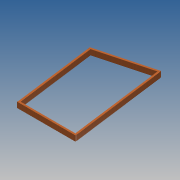
# Autodesk Inventor part: H7jp.E_UfaA-panelEframe
Saved by Autodesk Inventor 2014 SP1 (Build 180222100, 222)
## iProperties
Company: HERA
Created: 2015-04-29
Part Number: H7jp.E_UfaA-panelEframe
Material: Wood (Cherry)
Document SubType Name: Modeling
Designer: Dave
Mass: 16881.5 g
Surface Area: 18802.7 cm^2
Volume: 26796 cm^3
Density: 0.63 g/cm^3
Appearance: Cherry - Natural Low Gloss
Title: HERA Panel E frame
Author: Dave
Revision Number: A
Autodesk Inventor part; units mm, degrees
ref_plane "YZ Plane" through (0, 0, 0) normal (1, 0, 0) x (0, 1, 0)
ref_plane "XZ Plane" through (0, 0, 0) normal (0, 1, 0) x (-1, 0, 0)
ref_plane "XY Plane" through (0, 0, 0) normal (0, 0, 1) x (1, 0, 0)
sketch "Sketch1" plane through (0, 0, 0) normal (0, 1, 0) x (-1, 0, 0)
  line L0 (-1224.9972, -38) -> (-960.8978, -2044.0342)
  line L1 (-951.0627, -2080.7394) -> (232.1938, -1763.6868)
  line L2 (-955.895, -2082.0342) -> (274.105, -2082.0342) construction
  line L3 (227.191, -1725.6868) -> (5.0028, -38)
  line L4 (190.1691, -1735.6068) -> (-33.3251, -38)
  line L5 (-33.3251, -38) -> (-1186.6693, -38)
  line L6 (-1186.6693, -38) -> (-923.8759, -2034.1142)
  line L7 (-960.8978, -2044.0342) -> (-951.0627, -2080.7394)
  line L8 (-923.8759, -2034.1142) -> (190.1691, -1735.6068)
  line L9 (-1224.9972, -38) -> (-1224.9972, 0)
  line L10 (5.0028, -38) -> (5.0028, 0)
  line L11 (-1230, 0) -> (-1224.9972, 0) construction
  line L12 (5.0028, 0) -> (870, 0) construction
  line L13 (5.0028, 0) -> (-1224.9972, 0)
  line L14 (232.1938, -1763.6868) -> (237.0261, -1762.392)
  line L15 (227.191, -1725.6868) -> (237.0261, -1762.392)
  dimension "d1" = 2100
  dimension "d9" = 1230
  dimension "d10" = 15
  dimension "d12" = 38
  constraints: 32 end point, 4 perpendicular, 3 horizontal, 1 collinear, 1 parallel
  measures "d1" distance of L11.start L2.start
  measures "d9" distance of L2.start L1.end
  measures "d10" angle of L2 L1
  measures "d12" distance between parallel lines of L6 L0
extrude "Extrusion1" add sketch "Sketch1" along normal blind 114
sketch "Sketch2" plane through (0, 114, 0) normal (0, 1, 0) x (1, 0, 0)
  line L0 (33.3251, 38) -> (-190.1691, 1735.6068) projected
  line L1 (-227.191, 1725.6868) -> (-5.0028, 38) projected
  line L2 (1224.9972, 0) -> (1224.9972, 38) projected
  line L3 (960.8978, 2044.0342) -> (951.0627, 2080.7394) projected
  line L4 (-190.1691, 1735.6068) -> (-227.191, 1725.6868)
  line L5 (33.3251, 38) -> (-5.0028, 38)
  point P0 (0, 0)
  constraints: 4 end point, 2 perpendicular
extrude "Extrusion2" cut sketch "Sketch2" against normal blind 1
sketch "Sketch3" plane through (0, 114, 0) normal (0, 1, 0) x (1, 0, 0)
  line L0 (1224.9972, 0) -> (1224.9972, 38) projected
  line L1 (1224.9972, 38) -> (960.8978, 2044.0342) projected
  line L2 (960.8978, 2044.0342) -> (951.0627, 2080.7394) projected
  line L3 (951.0627, 2080.7394) -> (-237.0261, 1762.392) projected
  line L4 (-237.0261, 1762.392) -> (-227.191, 1725.6868) projected
  line L5 (-227.191, 1725.6868) -> (923.8759, 2034.1142) projected
  line L6 (923.8759, 2034.1142) -> (1186.6693, 38) projected
  line L7 (1186.6693, 38) -> (1224.9972, 38)
  line L8 (923.8759, 2034.1142) -> (960.8978, 2044.0342)
  point P0 (0, 0)
  constraints: 4 end point, 2 point on line, 1 collinear, 1 perpendicular
extrude "Extrusion3" cut sketch "Sketch3" against normal blind 1 contours L7 L6 L8 L1
body "Solid1"
